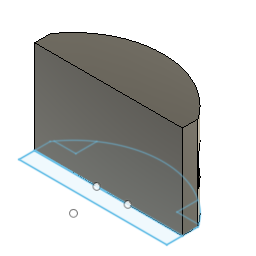
filler (Autodesk Fusion 360 design; units mm, degrees)
Autodesk Fusion 360 part; units mm, degrees
sketch "Sketch1" plane through (0, 0, 0) normal (0, 0, 1) x (1, 0, 0) in component "Component"
  arc A0 (19, 12) -> (0, 12) centre (9.5, 5.5) ccw
  line L0 (19, 10) -> (19, 12)
  line L1 (0, 10) -> (0, 12)
  line L2 (0, 10) -> (19, 10)
  line L3 (8, 10) -> (12, 10)
  line L4 (0.2158, 12.3047) -> (3, 12.3047)
  line L5 (3, 12.3047) -> (3, 15)
  line L6 (16.0158, 12.3047) -> (18.7842, 12.3047)
  line L7 (16.0158, 12.3047) -> (16.0158, 14.9891)
  line L8 (0, 10) -> (19, 10)
  line L9 (19, 10) -> (19, 8)
  line L10 (19, 8) -> (0, 8)
  line L11 (0, 8) -> (0, 10)
  dimension "d36" = 19
  constraint vertical L1
  constraint horizontal L2
  constraint horizontal L3
  constraint coincident L2 L3.start
  constraint coincident A0 L4.start
  constraint horizontal L4
  constraint coincident A0 L5.end
  constraint perpendicular L4 L5
  constraint horizontal L6
  constraint coincident A0 L6.end
  constraint coincident A0 L7.end
  constraint perpendicular L6 L7
  constraint horizontal L8
  constraint vertical L9
  constraint horizontal L10
  constraint vertical L11
  measures "d36" distance of L1.start L0.start
extrude "Extrude5" add sketch "Sketch1" along normal blind 12 contours A0 L0 L1 L2 L3 L4 L5 L6 L7 L8 | A0 L6 L7 | A0 L4 L5
extrude "Extrude6" cut sketch "Sketch1" along normal blind 8 contours A0 L6 L7
extrude "Extrude7" add sketch "Sketch1" along normal blind 4 contours A0 L6 L7
extrude "Extrude8" cut sketch "Sketch1" along normal blind 8 contours A0 L4 L5
extrude "Extrude9" add sketch "Sketch1" along normal blind 4 contours A0 L4 L5
extrude "Extrude3" [suppressed] in component "Component"
component "Component" placed x (1, 0, 0) y (0, 1, 0) z (0, 0, 1) at (0, 0, 0)
